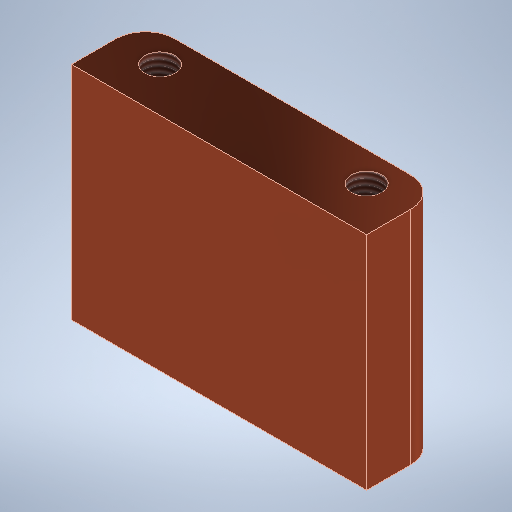
# Autodesk Inventor part: 02A
Saved by Autodesk Inventor 2025.1 (Build 291241000, 241)
## iProperties
Created: 2024-09-17
Part Number: 02A
Material: Aluminum 6061
Document SubType Name: Modeling
Designer: ffogue
Density: 2.7 g/cm^3
Appearance: Copper - Polished
Author: ffogue
Autodesk Inventor part; units mm, degrees
note: some values were not read from the file. Chosen so that the rebuilt part matches the saved one: direction of "Hole1".
ref_plane "YZ Plane" through (0, 0, 0) normal (1, 0, 0) x (0, 1, 0)
ref_plane "XZ Plane" through (0, 0, 0) normal (0, 1, 0) x (-1, 0, 0)
ref_plane "XY Plane" through (0, 0, 0) normal (0, 0, 1) x (1, 0, 0)
sketch "Sketch1" plane through (0, 0, 0) normal (0, 0, 1) x (1, 0, 0)
  line L0 (-20, 0) -> (20, 0)
  line L1 (20, 0) -> (20, 10)
  line L2 (20, 10) -> (-20, 10)
  line L3 (-20, 10) -> (-20, 0)
  point P0 (0, 0)
  point P1 (0, 0)
  dimension "d0" = 40
  dimension "d1" = 10
  constraints: 8 end point, 2 parallel, 1 coincident, 1 horizontal, 1 midpoint, 1 perpendicular
  measures "d0" distance of L1.end L2.end
  measures "d1" distance of L2.end L0.start
extrude "Extrusion1" add sketch "Sketch1" against normal blind 30
fillet "Fillet1" radius 4 2 edges at (20, 10, -15) (-20, 10, -15)
sketch "Sketch2" plane through (0, 0, 0) normal (0, 0, 1) x (1, 0, 0)
  arc A0 (-16, 10) -> (-20, 6) centre (-16, 6) ccw projected
  line L0 (-20, 6) -> (-20, 0) projected
  line L1 (-20, 0) -> (20, 0) projected
  line L2 (20, 0) -> (20, 6) projected
  arc A1 (20, 6) -> (16, 10) centre (16, 6) ccw projected
  line L3 (16, 10) -> (-16, 10) projected
  line L4 (-20, 0) -> (20, 0) projected
  point P0 (0, 0)
  point P1 (-14, 6)
  point P2 (14, 6)
  point P3 (0, 0)
  dimension "d12" = 28
  dimension "d13" = 14
  constraints: 2 horizontal alignment, 1 midpoint
  measures "d12" distance of point (14, 6) point (-14, 6)
  measures "d13" horizontal distance of point (0, 0) point (-14, 6)
hole "Hole1" at (-14, 6, 0) at (14, 6, 0) direction (0, 0, -1) diameter 4.134 depth 30 thread size "M5x0.8" class "6H" standard "ISO Metric profile"
equation "\"d13\" = 0.5 * d12"
body "Solid1"
